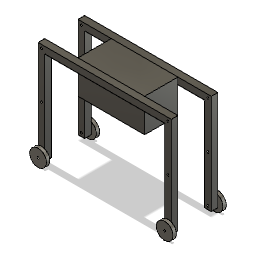
test_1 v3 (Autodesk Fusion 360 design; units mm, degrees)
part number: Configuration 1
Autodesk Fusion 360 part; units mm, degrees
sketch "Sketch1" plane through (0, 0, 0) normal (0, 0, 1) x (1, 0, 0)
  line L0 (0, 0) -> (200, 0)
  line L1 (200, 0) -> (200, 100)
  line L2 (200, 100) -> (0, 100)
  line L3 (0, 100) -> (0, 0)
  dimension "d1" = 200
  dimension "d2" = 100
  constraint horizontal L0
  constraint vertical L1
  constraint horizontal L2
  constraint vertical L3
  constraint coincident L0.start L3.end
  measures "d1" distance of L0.start L0.end
  measures "d2" distance of L0.start L2.end
extrude "Extrude1" add sketch "Sketch1" along normal blind 100 makes body 1
move_body "Move1" bodies 1 to x (1, 0, 0) y (0, 1, 0) z (0, 0, 1) at (0, 200, 0)
sketch "Sketch2" plane through (200, 0, 0) normal (1, 0, 0) x (0, 0, -1)
  line L0 (0, 200) -> (0, 300)
  line L1 (0, 300) -> (-100, 300)
  line L2 (-100, 300) -> (-100, 200)
  line L3 (-100, 200) -> (0, 200)
  line L4 (-100, 300) -> (-120, 300)
  line L5 (-120, 300) -> (-120, 280)
  line L6 (-120, 280) -> (-100, 280)
  line L7 (-100, 280) -> (-100, 300)
  line L8 (0, 300) -> (20, 300)
  line L9 (20, 300) -> (20, 280)
  line L10 (20, 280) -> (0, 280)
  line L11 (0, 280) -> (0, 300)
  dimension "d5" = 20
  dimension "d6" = 20
  dimension "d7" = 20
  dimension "d8" = 20
  constraint horizontal L4
  constraint vertical L5
  constraint horizontal L6
  constraint vertical L7
  constraint coincident L1.end L2.start
  constraint horizontal L8
  constraint vertical L9
  constraint horizontal L10
  constraint vertical L11
  constraint coincident L0.end L1.start
  measures "d5" distance of L1.end L4.end
  measures "d6" distance of L1.end L6.end
  measures "d7" distance of L0.end L8.end
  measures "d8" distance of L0.end L10.end
extrude "Extrude2" add sketch "Sketch2" against normal blind 200 separate body contours L0 L8 L9 L10 L11 | L2 L4 L5 L6 L7 makes body 2 at (133.3333, 280, 113.3333) makes body 3 at (133.3333, 286.6667, 0)
extrude "Extrude3" add 2 faces at (200, 293.3333, -6.6667) (200, 286.6667, 106.6667) along direction (1, 0, 0) blind 100 separate body on bodies 2 3 makes body 4 at (233.3333, 286.6667, 0) makes body 5 at (233.3333, 280, 113.3333)
extrude "Extrude4" add 2 faces at (0, 286.6667, 106.6667) (0, 293.3333, -6.6667) along direction (-1, 0, 0) blind 100 separate body on bodies 2 3 makes body 6 at (-33.3333, 280, 113.3333) makes body 7 at (-33.3333, 286.6667, 0)
combine "Combine1" operation add target body 7 tool bodies 4 3
combine "Combine2" operation add target body 6 tool bodies 5 2
sketch "Sketch3" plane through (0, 280, 0) normal (0, -1, 0) x (1, 0, 0)
  line L0 (300, 120) -> (-100, 120)
  line L1 (-100, 120) -> (-100, 100)
  line L2 (-100, 100) -> (300, 100)
  line L3 (300, 100) -> (300, 120)
  line L4 (-100, 100) -> (-80, 100)
  line L5 (-80, 100) -> (-80, 120)
  line L6 (-80, 120) -> (-100, 120)
  line L7 (-100, 120) -> (-100, 100)
  line L8 (-100, 0) -> (-80, 0)
  line L9 (-80, 0) -> (-80, -20)
  line L10 (-80, -20) -> (-100, -20)
  line L11 (-100, -20) -> (-100, 0)
  line L12 (300, 120) -> (280, 120)
  line L13 (280, 120) -> (280, 100)
  line L14 (280, 100) -> (300, 100)
  line L15 (300, 100) -> (300, 120)
  line L16 (300, 0) -> (280, 0)
  line L17 (280, 0) -> (280, -20)
  line L18 (280, -20) -> (300, -20)
  line L19 (300, -20) -> (300, 0)
  dimension "d15" = 20
  dimension "d16" = 20
  dimension "d17" = 20
  dimension "d18" = 20
  dimension "d19" = 20
  dimension "d20" = 20
  constraint horizontal L4
  constraint vertical L5
  constraint horizontal L6
  constraint vertical L7
  constraint coincident L1.end L2.start
  constraint horizontal L8
  constraint vertical L9
  constraint horizontal L10
  constraint vertical L11
  constraint horizontal L12
  constraint vertical L13
  constraint horizontal L14
  constraint vertical L15
  constraint coincident L0.start L3.end
  constraint horizontal L16
  constraint vertical L17
  constraint horizontal L18
  constraint vertical L19
  measures "d15" distance of L1.end L4.end
  measures "d16" distance of L1.end L0.end
  measures "d17" distance of L0.start L12.end
  measures "d18" distance of L0.start L2.end
  measures "d19" distance of L16.start L16.end
  measures "d20" distance of L16.start L18.end
extrude "Extrude5" add sketch "Sketch3" along normal blind 280 contours L0 L2 L3 L12 L13 L14 L15 | L0 L1 L2 L4 L5 L6 L7 | L8 L9 L10 L11 | L16 L17 L18 L19 bodies 6 7
sketch "Sketch4" plane through (0, 0, -20) normal (0, 0, -1) x (-1, 0, 0)
  line L0 (100, 0) -> (100, 300)
  line L1 (100, 300) -> (-300, 300)
  line L2 (-300, 300) -> (-300, 0)
  line L3 (-300, 0) -> (-280, 0)
  line L4 (-280, 0) -> (-280, 280)
  line L5 (-280, 280) -> (80, 280)
  line L6 (80, 280) -> (80, 0)
  line L7 (80, 0) -> (100, 0)
  circle A0 centre (-290, 10) radius 3
  circle A1 centre (90, 10) radius 3
  dimension "d23" = 6
  dimension "d24" = 6
  measures "d23" diameter of A0
  measures "d24" diameter of A1
extrude "Extrude6" cut sketch "Sketch4" against normal blind 160 contours A0 | A1 bodies 6 7
sketch "Sketch5" plane through (0, 0, -20) normal (0, 0, -1) x (-1, 0, 0)
sketch "Sketch6" plane through (0, 0, 0) normal (0, 0, 1) x (1, 0, 0)
  circle A0 centre (290, 290) radius 3
  dimension "d27" = 6
  measures "d27" diameter of A0
extrude "Extrude7" add sketch "Sketch6" along normal blind 140 and the other way blind 50 separate body makes body 8
copy_body "CopyPasteBodies1" bodies 8 makes body 9
move_body "Move2" bodies 9 to x (1, 0, 0) y (0, 1, 0) z (0, 0, 1) at (0, -140, 0)
copy_body "CopyPasteBodies2" bodies 9 makes body 10
move_body "Move3" bodies 10 to x (1, 0, 0) y (0, 1, 0) z (0, 0, 1) at (-380, 0, 0)
copy_body "CopyPasteBodies3" bodies 10 makes body 11
move_body "Move4" bodies 11 to x (1, 0, 0) y (0, 1, 0) z (0, 0, 1) at (0, 140, 0)
copy_body "CopyPasteBodies4" bodies 8 9 11 10 makes body 12 makes body 13 makes body 14 makes body 15
combine "Combine3" operation cut target body 7 tool bodies 10 11 8 13
combine "Combine4" operation cut target body 6 tool bodies 12 9 14 15
sketch "Sketch7" plane through (0, 200, 0) normal (0, -1, 0) x (1, 0, 0)
  line L0 (0, 0) -> (200, 0)
  line L1 (200, 0) -> (200, 100)
  line L2 (200, 100) -> (0, 100)
  line L3 (0, 100) -> (0, 0)
  circle A0 centre (40, 50) radius 20
  line L4 (170, 60) -> (190, 60)
  line L5 (190, 60) -> (190, 40)
  line L6 (190, 40) -> (170, 40)
  line L7 (170, 40) -> (170, 60)
  dimension "d32" = 40
  constraint horizontal L4
  constraint vertical L5
  constraint horizontal L6
  constraint vertical L7
  measures "d32" diameter of A0
extrude "Extrude8" add sketch "Sketch7" along normal blind 5 separate body contours A0 | L4 L5 L6 L7 makes body 16 at (39.9842, 200, 54.5345) makes body 17 at (176.6667, 200, 53.3333)
move_body "Move5" bodies 17 to x (1, 0, 0) y (0, 1, 0) z (0, 0, 1) at (-10, 0, 0)
sketch "Sketch8" plane through (0, 0, -20) normal (0, 0, -1) x (-1, 0, 0)
  circle A0 centre (-290, 150) radius 3
  circle A1 centre (-290, 290) radius 3
  circle A2 centre (90, 290) radius 3
  circle A3 centre (90, 150) radius 3
  circle A4 centre (-290, 10) radius 3
  circle A5 centre (90, 10) radius 3
  line L0 (100, 0) -> (100, 300)
  line L1 (100, 300) -> (-300, 300)
  line L2 (-300, 300) -> (-300, 0)
  line L3 (-300, 0) -> (-280, 0)
  line L4 (-280, 0) -> (-280, 280)
  line L5 (-280, 280) -> (80, 280)
  line L6 (80, 280) -> (80, 0)
  line L7 (80, 0) -> (100, 0)
  circle A6 centre (90, 10) radius 25
  circle A7 centre (-290, 10) radius 25
  dimension "d35" = 50
  dimension "d36" = 50
  constraint concentric A5 A6
  constraint concentric A4 A7
  measures "d35" diameter of A6
  measures "d36" diameter of A7
extrude "Extrude9" add sketch "Sketch8" along normal blind 10 separate body contours L0 L6 L7 A6 | L0 L6 L7 A6 | L2 L3 L4 A7 | L2 L3 L4 A7 makes body 18 at (-107.5624, 11.3911, -30) makes body 19 at (272.4376, 8.6089, -20)
copy_body "CopyPasteBodies5" bodies 19 18 makes body 20 makes body 21
copy_body "CopyPasteBodies6" bodies 21 20 makes body 22 makes body 23
move_body "Move6" bodies 22 23 to x (1, 0, 0) y (0, 1, 0) z (0, 0, 1) at (0, 0, 150)
